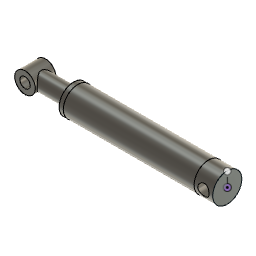
spargner v1 (Autodesk Fusion 360 design; units mm, degrees)
Autodesk Fusion 360 part; units mm, degrees
sketch "Sketch1" plane through (0, 0, 0) normal (1, 0, 0) x (0, 1, 0)
  circle A0 centre (0, 0) radius 3.1
  dimension "d1" = 6.2
  constraint coincident A0.centre origin
  measures "d1" diameter of A0
extrude "Extrude1" add sketch "Sketch1" against normal blind 4 makes body 1
extrude "Extrude1'" add 1 faces at (-4, -0.4599, 1.4057) along direction (-1, 0, 0) blind 28 separate body on bodies 1 makes body 2 in component "Component"
extrude "Extrude1''" add 1 faces at (-32, -0.4599, 1.4057) along direction (-1, 0, 0) blind 0.9 separate body on bodies 2 makes body 3 in component "Component'"
sketch "Sketch2" plane through (-32.9, 0, 0) normal (-1, 0, 0) x (0, -1, 0)
  circle A0 centre (0, 0) radius 3.1
  circle A1 centre (0, 0) radius 2.1
  dimension "d8" = 4.2
  constraint concentric A0 A1
  measures "d8" diameter of A1
extrude "Extrude2" add sketch "Sketch2" along normal blind 0.5 contours A1 bodies 3 in component "Component'"
sketch "Sketch3" plane through (-33.4, 0, 0) normal (-1, 0, 0) x (0, -1, 0)
  circle A0 centre (0, 0) radius 2.1
  circle A1 centre (0, 0) radius 1.8
  dimension "d11" = 3.6
  constraint concentric A0 A1
  measures "d11" diameter of A1
extrude "Extrude2'" add sketch "Sketch3" along normal blind 7.7 separate body contours A1 makes body 4
sketch "Sketch4" plane through (0, 0, 0) normal (0, 1, 0) x (1, 0, 0)
  circle A0 centre (-41.1047, 0.0084) radius 2.2
  dimension "d14" = 4.4
  measures "d14" diameter of A0
extrude "Extrude3" add sketch "Sketch4" along normal mid plane 4.4 bodies 4
sketch "Sketch5" plane through (0, 2.2, 0) normal (0, 1, 0) x (-1, 0, 0)
  circle A0 centre (41.1047, -0.0084) radius 2.2
  circle A1 centre (41.1047, -0.0084) radius 1.1
  dimension "d17" = 2.2
  constraint concentric A0 A1
  measures "d17" diameter of A1
extrude "Extrude4" cut sketch "Sketch5" against normal blind 5.607 contours A1 bodies 4
sketch "Sketch6" plane through (0, 0, 0) normal (0, 1, 0) x (1, 0, 0)
  circle A0 centre (-2, 0.0187) radius 1.2
  line L0 (0, -3.1) -> (0, 3.1)
  dimension "d20" = 2.4
  dimension "d21" = 2.4
  dimension "d22" = 2
  measures "d20" diameter of A0
  measures "d21" diameter of A0
  measures "d22" distance of A0.centre L0
extrude "Extrude5" cut sketch "Sketch6" along normal mid plane 13.01 bodies 1
sketch "Sketch7" plane through (0, 0, 0) normal (1, 0, 0) x (0, 1, 0)
sketch "Sketch8" plane through (0, 0, 0) normal (0, 0, 1) x (1, 0, 0)
  circle A0 centre (-5.0226, 4.9201) radius 1
  dimension "d25" = 2
  measures "d25" diameter of A0
sketch "Sketch9" plane through (0, 0, 0) normal (0, 0, -1) x (1, 0, 0)
  circle A0 centre (-5.0226, -4.9201) radius 1
  circle A1 centre (-5.0226, -4.9201) radius 0.8
  dimension "d28" = 1.6
  constraint concentric A0 A1
  measures "d28" diameter of A1
sketch "Sketch10" plane through (0, 0, -0.6) normal (0, 0, -1) x (1, 0, 0)
  circle A0 centre (-5.0226, -4.9201) radius 0.8
  circle A1 centre (-5.0226, -4.9201) radius 0.6
  dimension "d31" = 1.2
  constraint concentric A0 A1
  measures "d31" diameter of A1
sketch "Sketch11" plane through (0, 0, 0) normal (0, 0, -1) x (1, 0, 0)
  circle A0 centre (-5.0226, -4.9201) radius 0.8
  circle A1 centre (-5.0226, -4.9201) radius 1
  circle A2 centre (-5.0226, -4.9201) radius 1.2
  dimension "d34" = 2.4
  constraint concentric A0 A2
  measures "d34" diameter of A2
sketch "Sketch12" plane through (0, 0, -0.6) normal (0, 0, -1) x (1, 0, 0)
  circle A0 centre (-5.0226, -4.9201) radius 1.2
  line L0 (-5.0985, -4.0295) -> (-5.0985, -3.6215)
  line L1 (-4.8985, -4.028) -> (-4.8985, -3.6403)
  line L2 (-4.9985, -4.9971) -> (-4.9985, -3.4779) construction
  line L3 (-5.1941, -3.8971) -> (-4.7341, -3.8971)
  circle A1 centre (-5.0226, -4.9201) radius 0.8
  dimension "d37" = 0.1
  dimension "d38" = 0.1
  dimension "d41" = 1.1
  constraint vertical L0
  constraint vertical L1
  constraint horizontal L3
  measures "d37" distance of L0 L2
  measures "d38" distance of L1 L2
  measures "d41" distance of L2.start L3
extrude "Extrude10" add sketch "Sketch12" against normal blind 0.6 separate body contours A0 L0 L1 L3 picked at (-4.9874, -3.8385) makes body 5
sketch "Sketch13" plane through (0, 0, -0.6) normal (0, 0, -1) x (1, 0, 0)
  line L0 (-4.8985, -3.8971) -> (-4.8985, -3.7265)
  arc A0 (-4.8985, -3.7265) -> (-5.0985, -3.7225) centre (-5.0226, -4.9201) ccw
  line L1 (-5.0985, -3.7225) -> (-5.0985, -3.8971)
  line L2 (-5.0985, -3.8971) -> (-4.8985, -3.8971)
  line L3 (-5.0226, -4.9201) -> (-4.9575, -5.4988)
  arc A1 (-5.3142, -3.7561) -> (-5.5035, -3.8207) centre (-5.0226, -4.9201) ccw
  line L4 (-5.2559, -3.9163) -> (-5.3142, -3.7561)
  line L5 (-5.4438, -3.9847) -> (-5.2559, -3.9163)
  line L6 (-5.5035, -3.8207) -> (-5.4438, -3.9847)
  arc A2 (-5.6948, -3.926) -> (-5.8506, -4.0515) centre (-5.0226, -4.9201) ccw
  line L7 (-5.5851, -4.0567) -> (-5.6948, -3.926)
  line L8 (-5.7383, -4.1852) -> (-5.5851, -4.0567)
  line L9 (-5.8506, -4.0515) -> (-5.7383, -4.1852)
  arc A3 (-5.9942, -4.2158) -> (-6.0977, -4.387) centre (-5.0226, -4.9201) ccw
  line L10 (-5.8465, -4.3011) -> (-5.9942, -4.2158)
  line L11 (-5.9465, -4.4743) -> (-5.8465, -4.3011)
  line L12 (-6.0977, -4.387) -> (-5.9465, -4.4743)
  arc A4 (-6.1765, -4.5906) -> (-6.2152, -4.7869) centre (-5.0226, -4.9201) ccw
  line L13 (-6.0085, -4.6202) -> (-6.1765, -4.5906)
  line L14 (-6.0433, -4.8172) -> (-6.0085, -4.6202)
  line L15 (-6.2152, -4.7869) -> (-6.0433, -4.8172)
  arc A5 (-6.2196, -5.0051) -> (-6.1888, -5.2028) centre (-5.0226, -4.9201) ccw
  line L16 (-6.0516, -4.9755) -> (-6.2196, -5.0051)
  line L17 (-6.0169, -5.1725) -> (-6.0516, -4.9755)
  line L18 (-6.1888, -5.2028) -> (-6.0169, -5.1725)
  arc A6 (-6.1183, -5.4094) -> (-6.0218, -5.5846) centre (-5.0226, -4.9201) ccw
  line L19 (-5.9706, -5.3241) -> (-6.1183, -5.4094)
  line L20 (-5.8706, -5.4973) -> (-5.9706, -5.3241)
  line L21 (-6.0218, -5.5846) -> (-5.8706, -5.4973)
  arc A7 (-5.8849, -5.7546) -> (-5.7343, -5.8863) centre (-5.0226, -4.9201) ccw
  line L22 (-5.7752, -5.624) -> (-5.8849, -5.7546)
  line L23 (-5.622, -5.7525) -> (-5.7752, -5.624)
  line L24 (-5.7343, -5.8863) -> (-5.622, -5.7525)
  arc A8 (-5.5474, -5.9992) -> (-5.3609, -6.0714) centre (-5.0226, -4.9201) ccw
  line L25 (-5.4891, -5.839) -> (-5.5474, -5.9992)
  line L26 (-5.3012, -5.9074) -> (-5.4891, -5.839)
  line L27 (-5.3609, -6.0714) -> (-5.3012, -5.9074)
  arc A9 (-5.1467, -6.1137) -> (-4.9467, -6.1177) centre (-5.0226, -4.9201) ccw
  line L28 (-5.1467, -5.9431) -> (-5.1467, -6.1137)
  line L29 (-4.9467, -5.9431) -> (-5.1467, -5.9431)
  line L30 (-4.9467, -6.1177) -> (-4.9467, -5.9431)
  arc A10 (-4.731, -6.0841) -> (-4.5417, -6.0195) centre (-5.0226, -4.9201) ccw
  line L31 (-4.7893, -5.9238) -> (-4.731, -6.0841)
  line L32 (-4.6014, -5.8554) -> (-4.7893, -5.9238)
  line L33 (-4.5417, -6.0195) -> (-4.6014, -5.8554)
  arc A11 (-4.3505, -5.9142) -> (-4.1947, -5.7887) centre (-5.0226, -4.9201) ccw
  line L34 (-4.4601, -5.7835) -> (-4.3505, -5.9142)
  line L35 (-4.3069, -5.655) -> (-4.4601, -5.7835)
  line L36 (-4.1947, -5.7887) -> (-4.3069, -5.655)
  arc A12 (-4.051, -5.6243) -> (-3.9475, -5.4532) centre (-5.0226, -4.9201) ccw
  line L37 (-4.1987, -5.5391) -> (-4.051, -5.6243)
  line L38 (-4.0987, -5.3659) -> (-4.1987, -5.5391)
  line L39 (-3.9475, -5.4532) -> (-4.0987, -5.3659)
  arc A13 (-3.8687, -5.2496) -> (-3.83, -5.0533) centre (-5.0226, -4.9201) ccw
  line L40 (-4.0367, -5.2199) -> (-3.8687, -5.2496)
  line L41 (-4.002, -5.023) -> (-4.0367, -5.2199)
  line L42 (-3.83, -5.0533) -> (-4.002, -5.023)
  arc A14 (-3.8256, -4.835) -> (-3.8564, -4.6374) centre (-5.0226, -4.9201) ccw
  line L43 (-3.9936, -4.8647) -> (-3.8256, -4.835)
  line L44 (-4.0283, -4.6677) -> (-3.9936, -4.8647)
  line L45 (-3.8564, -4.6374) -> (-4.0283, -4.6677)
  arc A15 (-3.9269, -4.4308) -> (-4.0234, -4.2556) centre (-5.0226, -4.9201) ccw
  line L46 (-4.0746, -4.5161) -> (-3.9269, -4.4308)
  line L47 (-4.1746, -4.3429) -> (-4.0746, -4.5161)
  line L48 (-4.0234, -4.2556) -> (-4.1746, -4.3429)
  arc A16 (-4.1603, -4.0855) -> (-4.311, -3.9539) centre (-5.0226, -4.9201) ccw
  line L49 (-4.27, -4.2162) -> (-4.1603, -4.0855)
  line L50 (-4.4232, -4.0876) -> (-4.27, -4.2162)
  line L51 (-4.311, -3.9539) -> (-4.4232, -4.0876)
  arc A17 (-4.4978, -3.841) -> (-4.6843, -3.7688) centre (-5.0226, -4.9201) ccw
  line L52 (-4.5561, -4.0012) -> (-4.4978, -3.841)
  line L53 (-4.744, -3.9328) -> (-4.5561, -4.0012)
  line L54 (-4.6843, -3.7688) -> (-4.744, -3.9328)
  dimension "d45" = 360
  constraint coincident A0.centre L3.start
sketch "Sketch14" plane through (0, 0, 0) normal (1, 0, 0) x (0, 1, 0)
  circle A0 centre (0, 0) radius 3.1
sketch "Sketch15" plane through (0, 0, 0) normal (1, 0, 0) x (0, 1, 0)
ref_plane "WorkPlane1" through (-6.4, 0, 0) normal (1, 0, 0) x (0, 1, 0)
sketch "Sketch16" plane through (-6.4, 0, 0) normal (1, 0, 0) x (0, 1, 0)
sketch "Sketch17" plane through (0, 0, 0) normal (1, 0, 0) x (0, 1, 0)
  line L0 (0, 0) -> (0, 3.0141) construction
  constraint coincident L0.start origin
  constraint vertical L0
sketch "Sketch18" plane through (0, 0, 0) normal (0, 0, 1) x (1, 0, 0)
component "Component" placed x (1, 0, 0) y (0, 1, 0) z (0, 0, 1) at (0, 0, 0)
component "Component'" placed x (1, 0, 0) y (0, 1, 0) z (0, 0, 1) at (0, 0, 0)
